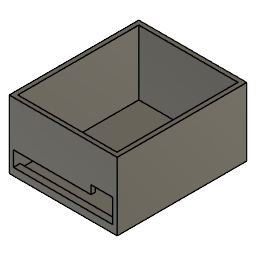
satelitenas (Autodesk Fusion 360 design; units mm, degrees)
Autodesk Fusion 360 part; units mm, degrees
sketch "Sketch1" plane through (0, 0, 0) normal (0, 0, 1) x (1, 0, 0)
  line L0 (-71.12, 30.48) -> (106.68, 30.48)
  line L1 (106.68, 30.48) -> (106.68, -102.87)
  line L2 (106.68, -102.87) -> (-71.12, -102.87)
  line L3 (-71.12, -102.87) -> (-71.12, 30.48)
  dimension "d1" = 177.8
  dimension "d2" = 133.35
  constraint horizontal L0
  constraint vertical L1
  constraint horizontal L2
  constraint vertical L3
  measures "d1" distance of L0.start L0.end
  measures "d2" distance of L0.start L2.end
sketch "Sketch2" plane through (0, 0, 0) normal (0, 0, 1) x (1, 0, 0)
  line L0 (-71.12, 30.48) -> (119.38, 30.48)
  line L1 (119.38, 30.48) -> (119.38, -115.57)
  line L2 (119.38, -115.57) -> (-71.12, -115.57)
  line L3 (-71.12, -115.57) -> (-71.12, 30.48)
  dimension "d23" = 146.05
  constraint horizontal L0
  constraint vertical L1
  constraint horizontal L2
  constraint vertical L3
  measures "d23" distance of L0.start L2.end
sketch "Sketch3" plane through (-71.12, 0, 0) normal (-1, 0, 0) x (0, -1, 0)
  line L0 (102.87, 0) -> (115.57, 0)
  line L1 (115.57, 0) -> (115.57, 114.3)
  line L2 (115.57, 114.3) -> (102.87, 114.3)
  line L3 (88.9, 5.08) -> (38.1, 5.08)
  line L4 (38.1, 5.08) -> (38.1, 17.78)
  line L5 (38.1, 17.78) -> (88.9, 17.78)
  line L6 (88.9, 17.78) -> (88.9, 5.08)
  line L7 (102.87, 114.3) -> (102.87, 0)
  dimension "d26" = 12.7
  constraint horizontal L3
  constraint vertical L4
  constraint horizontal L5
  constraint vertical L6
  measures "d26" distance of L3.start L5.end
sketch "Sketch4" plane through (0, 0, 0) normal (0, 0, 1) x (1, 0, 0)
  line L0 (-76.2, 63.5) -> (-19.05, 63.5)
  line L1 (-19.05, 63.5) -> (-19.05, -6.35)
  line L2 (-19.05, -6.35) -> (-76.2, -6.35)
  line L3 (-76.2, -6.35) -> (-76.2, 63.5)
  dimension "d29" = 57.15
  dimension "d30" = 69.85
  constraint horizontal L0
  constraint vertical L1
  constraint horizontal L2
  constraint vertical L3
  measures "d29" distance of L0.start L0.end
  measures "d30" distance of L0.start L2.end
extrude "Extrude13" add sketch "Sketch4" along normal blind 40.005
sketch "Sketch5" plane through (0, 0, 40.005) normal (0, 0, 1) x (-1, 0, 0)
  line L0 (76.2, 6.35) -> (19.05, 6.35)
  line L1 (19.05, 6.35) -> (19.05, -63.5)
  line L2 (19.05, -63.5) -> (76.2, -63.5)
  line L3 (76.2, -63.5) -> (76.2, 6.35)
  line L4 (73.66, -60.96) -> (21.7077, -60.96)
  line L5 (21.7077, -60.96) -> (21.7077, 3.8213)
  line L6 (21.7077, 3.8213) -> (73.66, 3.8213)
  line L7 (73.66, 3.8213) -> (73.66, -60.96)
  constraint horizontal L4
  constraint vertical L5
  constraint horizontal L6
  constraint vertical L7
extrude "Extrude14" cut sketch "Sketch5" against normal blind 38.1 contours L4 L5 L6 L7
sketch "Sketch6" plane through (0, -6.35, 0) normal (0, -1, 0) x (1, 0, 0)
  line L0 (-76.2, 0) -> (-19.05, 0)
  line L1 (-19.05, 0) -> (-19.05, 40.005)
  line L2 (-19.05, 40.005) -> (-76.2, 40.005)
  line L3 (-76.2, 40.005) -> (-76.2, 0)
  line L4 (-22.86, 2.54) -> (-73.66, 2.54)
  line L5 (-73.66, 2.54) -> (-73.66, 15.24)
  line L6 (-73.66, 15.24) -> (-22.86, 15.24)
  line L7 (-22.86, 15.24) -> (-22.86, 2.54)
  dimension "d35" = 50.8
  dimension "d36" = 12.7
  constraint horizontal L4
  constraint vertical L5
  constraint horizontal L6
  constraint vertical L7
  measures "d35" distance of L4.start L4.end
  measures "d36" distance of L4.start L6.end
extrude "Extrude15" cut sketch "Sketch6" against normal blind 19.9898 contours L4 L5 L6 L7
extrude "Extrude16" cut 1 faces at (-56.7267, -4.6642, 2.54) along direction (0, 0, -1) blind 0.635
extrude "Extrude17" add 1 faces at (-39.7933, -4.6642, 15.24) along direction (0, 0, -1) blind 1.905
extrude "Extrude18" add 1 faces at (-19.05, 40.2167, 13.335) along direction (1, 0, 0) blind 6.35
extrude "Extrude19" cut 1 faces at (-21.7077, 17.7724, 27.305) along direction (1, 0, 0) blind 6.35
extrude "Extrude20" cut 1 faces at (-22.86, -4.6642, 5.715) along direction (1, 0, 0) blind 7.62
extrude "Extrude21" add 1 faces at (-15.24, -4.6642, 5.715) along direction (-1, 0, 0) blind 0.127
extrude "Extrude22" add 1 faces at (-55.0333, 63.5, 13.335) along direction (0, 1, 0) blind 6.35
extrude "Extrude23" cut 1 faces at (-54.2259, 60.96, 27.305) along direction (0, 1, 0) blind 6.35
sketch "Sketch7" plane through (0, 0, 1.905) normal (0, 0, 1) x (-1, 0, 0)
  line L0 (15.367, 6.35) -> (15.367, 3.8213)
  line L1 (15.367, 3.8213) -> (15.3577, 3.8213)
  line L2 (15.3577, 3.8213) -> (15.3577, -67.31)
  line L3 (15.3577, -67.31) -> (73.66, -67.31)
  line L4 (73.66, -67.31) -> (73.66, 6.35)
  line L5 (73.66, 6.35) -> (15.367, 6.35)
  line L6 (73.66, 6.35) -> (15.367, 6.35)
  line L7 (15.367, 6.35) -> (15.367, 2.4713)
  line L8 (15.367, 2.4713) -> (73.66, 2.4713)
  line L9 (73.66, 2.4713) -> (73.66, 6.35)
  constraint horizontal L6
  constraint vertical L7
  constraint horizontal L8
  constraint vertical L9
  constraint coincident L4.end L5.start
extrude "Extrude24" add sketch "Sketch7" along normal blind 2.54 contours L0 L4 L5 L6 L7 L8 L9
sketch "Sketch8" plane through (0, 0, 13.335) normal (0, 0, -1) x (1, 0, 0)
  line L0 (-15.367, 3.8213) -> (-15.367, 6.35)
  line L1 (-15.367, 6.35) -> (-73.66, 6.35)
  line L2 (-73.66, 6.35) -> (-73.66, 3.8213)
  line L3 (-73.66, 3.8213) -> (-15.367, 3.8213)
  line L4 (-15.367, 3.8213) -> (-28.067, 3.8213)
  line L5 (-28.067, 3.8213) -> (-28.067, 6.35)
  line L6 (-28.067, 6.35) -> (-15.367, 6.35)
  line L7 (-15.367, 6.35) -> (-15.367, 3.8213)
  dimension "d57" = 12.7
  constraint horizontal L4
  constraint vertical L5
  constraint horizontal L6
  constraint vertical L7
  constraint coincident L0.start L3.end
  measures "d57" distance of L0.start L4.end
extrude "Extrude25" cut sketch "Sketch8" against normal blind 5.0038 contours L0 L1 L3 L4 L5 L6 L7
